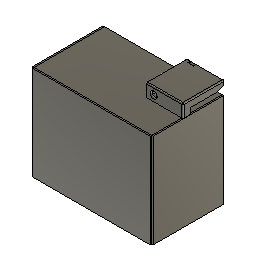
Pantry Working_ (Autodesk Fusion 360 design; units mm, degrees)
Autodesk Fusion 360 part; units mm, degrees
sketch "Sketch1" plane through (0, 0, 0) normal (0, 0, 1) x (1, 0, 0)
  line L0 (0, 0) -> (6.35, 0)
  line L1 (6.35, 0) -> (6.35, 300)
  line L2 (6.35, 300) -> (0, 300)
  line L3 (0, 300) -> (0, 0)
  line L4 (6.35, 0) -> (506.35, 0)
  line L5 (506.35, 0) -> (506.35, -6.35)
  line L6 (506.35, -6.35) -> (6.35, -6.35)
  line L7 (6.35, -6.35) -> (6.35, 0)
  line L8 (506.35, 0) -> (512.7, 0)
  line L9 (512.7, 0) -> (512.7, 300)
  line L10 (512.7, 300) -> (506.35, 300)
  line L11 (506.35, 300) -> (506.35, 0)
  line L12 (6.35, 300) -> (506.35, 300)
  dimension "d1" = 6.35
  dimension "d2" = 300
  dimension "d3" = 500
  dimension "d4" = 6.35
  dimension "d5" = 6.35
  dimension "d6" = 300
  constraint horizontal L0
  constraint vertical L1
  constraint horizontal L2
  constraint vertical L3
  constraint coincident L0.start L3.end
  constraint horizontal L4
  constraint vertical L5
  constraint horizontal L6
  constraint vertical L7
  constraint horizontal L8
  constraint vertical L9
  constraint horizontal L10
  constraint vertical L11
  measures "d1" distance of L0.start L0.end
  measures "d2" distance of L0.start L2.end
  measures "d3" distance of L0.end L4.end
  measures "d4" distance of L0.end L6.end
  measures "d5" distance of L4.end L8.end
  measures "d6" distance of L4.end L10.end
extrude "Extrude1" add sketch "Sketch1" along normal blind 400 contours L0 L1 L2 L3 | L4 L5 L6 L7 | L8 L9 L10 L11 makes body 1 at (0, 200, 133.3333)
extrude "Extrude2" add sketch "Sketch1" along normal blind 12.7 separate body contours L1 L4 L11 L12 makes body 2
ref_plane "WorkPlane1" through (0, 0, 220) normal (0, 0, 1) x (1, 0, 0)
sketch "Sketch2" plane through (0, 0, 220) normal (0, 0, 1) x (1, 0, 0)
  line L0 (6.35, 0) -> (506.35, 0)
  line L1 (506.35, 0) -> (506.35, 300)
  line L2 (506.35, 300) -> (6.35, 300)
  line L3 (6.35, 300) -> (6.35, 0)
  line L4 (6.35, 0) -> (506.35, 0)
  line L5 (506.35, 0) -> (506.35, 150)
  line L6 (506.35, 150) -> (6.35, 150)
  line L7 (6.35, 150) -> (6.35, 0)
  line L8 (506.35, 150) -> (406.35, 150)
  line L9 (406.35, 150) -> (406.35, 300)
  line L10 (406.35, 300) -> (506.35, 300)
  line L11 (506.35, 300) -> (506.35, 150)
  line L12 (6.35, 150) -> (106.35, 150)
  line L13 (106.35, 150) -> (106.35, 300)
  line L14 (106.35, 300) -> (6.35, 300)
  line L15 (6.35, 300) -> (6.35, 150)
  dimension "d12" = 500
  dimension "d13" = 150
  dimension "d14" = 100
  dimension "d15" = 150
  dimension "d16" = 100
  dimension "d17" = 150
  constraint horizontal L4
  constraint vertical L5
  constraint horizontal L6
  constraint vertical L7
  constraint coincident L0.start L3.end
  constraint horizontal L8
  constraint vertical L9
  constraint horizontal L10
  constraint vertical L11
  constraint horizontal L12
  constraint vertical L13
  constraint horizontal L14
  constraint vertical L15
  measures "d12" distance of L0.start L0.end
  measures "d13" distance of L0.start L6.end
  measures "d14" distance of L5.end L8.end
  measures "d15" distance of L5.end L1.end
  measures "d16" distance of L6.end L12.end
  measures "d17" distance of L6.end L2.end
extrude "Extrude3" add sketch "Sketch2" along normal blind 12.7 separate body contours L0 L1 L3 L4 L5 L6 L7 L8 L12 | L2 L3 L6 L12 L13 L14 L15 | L1 L2 L6 L8 L9 L10 L11 makes body 3
ref_plane "WorkPlane2" through (0, 0, 400) normal (0, 0, 1) x (1, 0, 0)
sketch "Sketch3" plane through (0, 0, 400) normal (0, 0, 1) x (1, 0, 0)
  line L0 (6.35, 0) -> (506.35, 0)
  line L1 (506.35, 0) -> (506.35, 300)
  line L2 (506.35, 300) -> (6.35, 300)
  line L3 (6.35, 300) -> (6.35, 0)
extrude "Extrude4" add sketch "Sketch3" against normal blind 12.7 separate body makes body 4
sketch "Sketch4" plane through (0, 0, 232.7) normal (0, 0, 1) x (-1, 0, 0)
  line L0 (-406.35, -150) -> (-106.35, -150)
  line L1 (-106.35, -150) -> (-106.35, -300)
  line L2 (-106.35, -300) -> (-6.35, -300)
  line L3 (-6.35, -300) -> (-6.35, 0)
  line L4 (-6.35, 0) -> (-506.35, 0)
  line L5 (-506.35, 0) -> (-506.35, -300)
  line L6 (-506.35, -300) -> (-406.35, -300)
  line L7 (-406.35, -300) -> (-406.35, -150)
  line L8 (-406.35, -150) -> (-421.35, -150)
  line L9 (-421.35, -150) -> (-421.35, -175)
  line L10 (-421.35, -175) -> (-406.35, -175)
  line L11 (-406.35, -175) -> (-406.35, -150)
  line L12 (-406.35, -150) -> (-381.35, -150)
  line L13 (-381.35, -150) -> (-381.35, -135)
  line L14 (-381.35, -135) -> (-406.35, -135)
  line L15 (-406.35, -135) -> (-406.35, -150)
  line L16 (-381.35, -150) -> (-406.35, -175)
  line L17 (-406.35, -135) -> (-421.35, -135)
  line L18 (-421.35, -135) -> (-421.35, -150)
  line L19 (-421.35, -150) -> (-406.35, -150)
  line L20 (-406.35, -150) -> (-406.35, -135)
  dimension "d23" = 15
  dimension "d24" = 25
  dimension "d25" = 25
  dimension "d26" = 15
  constraint horizontal L8
  constraint vertical L9
  constraint horizontal L10
  constraint vertical L11
  constraint coincident L0.start L7.end
  constraint horizontal L12
  constraint vertical L13
  constraint horizontal L14
  constraint vertical L15
  constraint horizontal L17
  constraint vertical L18
  constraint horizontal L19
  constraint vertical L20
  measures "d23" distance of L0.start L8.end
  measures "d24" distance of L0.start L10.end
  measures "d25" distance of L0.start L12.end
  measures "d26" distance of L0.start L14.end
extrude "Extrude5" add sketch "Sketch4" along normal blind 5 separate body contours L0 L12 L13 L14 L15 L20 | L0 L7 L11 L12 L16 | L7 L8 L9 L10 L11 L19 | L8 L15 L17 L18 L19 L20 makes body 5
extrude "Extrude7" add 1 faces at (403.0167, 158.3333, 232.7) along direction (0, 0, -1) blind 17.7 on bodies 5 bodies 5
extrude "Extrude8" cut sketch "Sketch4" against normal blind 12.7 contours L0 L12 L13 L14 L15 L20 | L7 L8 L9 L10 L11 L19 | L8 L15 L17 L18 L19 L20 bodies 5
fillet "Fillet1" radius 10 6 edges at (421.35, 175, 235.2) (421.35, 135, 235.2) (421.35, 175, 217.5) (421.35, 135, 217.5) (381.35, 135, 217.5) (381.35, 135, 235.2) on bodies 5
copy_body "Body->Comp1" bodies 1 removing the originals makes body 6 in component "walls"
copy_body "Body->Comp2" bodies 2 removing the originals makes body 7 in component "bottom"
copy_body "Body->Comp3" bodies 4 removing the originals makes body 8 in component "top"
copy_body "Body->Comp4" bodies 3 removing the originals makes body 9 in component "inner shelf"
copy_body "Body->Comp5" bodies 5 removing the originals makes body 10 in component "corner support"
sketch "Sketch5" plane through (0, 0, 400) normal (0, 0, 1) x (-1, 0, 0)
  line L0 (-6.35, -300) -> (-6.35, 0)
  line L1 (-6.35, 0) -> (-506.35, 0)
  line L2 (-506.35, 0) -> (-506.35, -300)
  line L3 (-506.35, -300) -> (-6.35, -300)
  line L4 (-506.35, -300) -> (-306.35, -300)
  line L5 (-306.35, -300) -> (-306.35, -100)
  line L6 (-306.35, -100) -> (-506.35, -100)
  line L7 (-506.35, -100) -> (-506.35, -300)
  line L8 (-506.35, -300) -> (-426.35, -300)
  line L9 (-426.35, -300) -> (-426.35, -195)
  line L10 (-426.35, -195) -> (-506.35, -195)
  line L11 (-506.35, -195) -> (-506.35, -300)
  line L12 (-426.35, -300) -> (-416.35, -300)
  line L13 (-416.35, -300) -> (-416.35, -195)
  line L14 (-416.35, -195) -> (-426.35, -195)
  line L15 (-426.35, -195) -> (-426.35, -300)
  line L16 (-416.35, -300) -> (-356.35, -300)
  line L17 (-356.35, -300) -> (-356.35, -133)
  line L18 (-356.35, -133) -> (-416.35, -133)
  line L19 (-416.35, -133) -> (-416.35, -300)
  line L20 (-356.35, -133) -> (-351.35, -133)
  line L21 (-351.35, -133) -> (-351.35, -300)
  line L22 (-351.35, -300) -> (-356.35, -300)
  line L23 (-356.35, -300) -> (-356.35, -133)
  line L24 (-351.35, -300) -> (-511.35, -300)
  line L25 (-511.35, -300) -> (-511.35, -305)
  line L26 (-511.35, -305) -> (-351.35, -305)
  line L27 (-351.35, -305) -> (-351.35, -300)
  line L28 (-511.35, -300) -> (-506.35, -300)
  line L29 (-506.35, -300) -> (-506.35, -133)
  line L30 (-506.35, -133) -> (-511.35, -133)
  line L31 (-511.35, -133) -> (-511.35, -300)
  line L32 (-351.35, -133) -> (-511.35, -133)
  line L33 (-511.35, -133) -> (-511.35, -128)
  line L34 (-511.35, -128) -> (-351.35, -128)
  line L35 (-351.35, -128) -> (-351.35, -133)
  dimension "d41" = 200
  dimension "d42" = 200
  dimension "d43" = 80
  dimension "d44" = 105
  dimension "d45" = 10
  dimension "d46" = 105
  dimension "d47" = 60
  dimension "d48" = 167
  dimension "d49" = 5
  dimension "d50" = 167
  dimension "d51" = 160
  dimension "d52" = 5
  dimension "d53" = 5
  dimension "d54" = 167
  dimension "d55" = 160
  dimension "d56" = 5
  constraint horizontal L4
  constraint vertical L5
  constraint horizontal L6
  constraint vertical L7
  constraint coincident L2.end L3.start
  constraint horizontal L8
  constraint vertical L9
  constraint horizontal L10
  constraint vertical L11
  constraint horizontal L12
  constraint vertical L13
  constraint horizontal L14
  constraint vertical L15
  constraint horizontal L16
  constraint vertical L17
  constraint horizontal L18
  constraint vertical L19
  constraint horizontal L20
  constraint vertical L21
  constraint horizontal L22
  constraint vertical L23
  constraint horizontal L24
  constraint vertical L25
  constraint horizontal L26
  constraint vertical L27
  constraint horizontal L28
  constraint vertical L29
  constraint horizontal L30
  constraint vertical L31
  constraint horizontal L32
  constraint vertical L33
  constraint horizontal L34
  constraint vertical L35
  measures "d41" distance of L2.end L4.end
  measures "d42" distance of L2.end L6.end
  measures "d43" distance of L2.end L8.end
  measures "d44" distance of L2.end L10.end
  measures "d45" distance of L8.end L12.end
  measures "d46" distance of L8.end L9.end
  measures "d47" distance of L12.end L16.end
  measures "d48" distance of L12.end L18.end
  measures "d49" distance of L17.end L20.end
  measures "d50" distance of L17.end L16.end
  measures "d51" distance of L21.end L24.end
  measures "d52" distance of L21.end L26.end
  measures "d53" distance of L24.end L2.end
  measures "d54" distance of L24.end L30.end
  measures "d55" distance of L20.end L30.end
  measures "d56" distance of L20.end L34.end
extrude "Extrude9" add sketch "Sketch5" along normal blind 55 separate body contours L3 L4 L8 L12 L16 L22 L24 L25 L26 L27 L28 | L3 L4 L17 L20 L21 L22 L23 L24 L32 | L2 L7 L18 L20 L32 L34 L35 | L2 L7 L30 L32 L33 L34 | L2 L7 L11 L24 L28 L29 L30 L31 L32 makes body 11
sketch "Sketch6" plane through (511.35, 0, 0) normal (1, 0, 0) x (0, 1, 0)
  line L0 (128, 400) -> (305, 400)
  line L1 (305, 400) -> (305, 455)
  line L2 (305, 455) -> (128, 455)
  line L3 (128, 455) -> (128, 400)
  line L4 (305, 400) -> (160, 400)
  line L5 (160, 400) -> (160, 425)
  line L6 (160, 425) -> (305, 425)
  line L7 (305, 425) -> (305, 400)
  dimension "d59" = 145
  dimension "d60" = 25
  constraint horizontal L4
  constraint vertical L5
  constraint horizontal L6
  constraint vertical L7
  constraint coincident L0.end L1.start
  measures "d59" distance of L0.end L4.end
  measures "d60" distance of L0.end L6.end
sketch "Sketch7" plane through (0, 305, 0) normal (0, 1, 0) x (-1, 0, 0)
  line L0 (-511.35, 400) -> (-351.35, 400)
  line L1 (-351.35, 400) -> (-351.35, 455)
  line L2 (-351.35, 455) -> (-511.35, 455)
  line L3 (-511.35, 455) -> (-511.35, 400)
  line L4 (-511.35, 400) -> (-461.35, 400)
  line L5 (-461.35, 400) -> (-461.35, 435)
  line L6 (-461.35, 435) -> (-511.35, 435)
  line L7 (-511.35, 435) -> (-511.35, 400)
  line L8 (-351.35, 400) -> (-376.35, 400) construction
  line L9 (-376.35, 400) -> (-389.35, 400)
  line L10 (-389.35, 400) -> (-389.35, 422)
  line L11 (-389.35, 422) -> (-376.35, 422)
  line L12 (-376.35, 422) -> (-376.35, 400)
  line L13 (-445, 440) -> (-420, 440)
  line L14 (-420, 440) -> (-420, 425)
  line L15 (-420, 425) -> (-445, 425)
  line L16 (-445, 425) -> (-445, 440)
  dimension "d61" = 50
  dimension "d62" = 35
  dimension "d63" = 25
  dimension "d64" = 13
  dimension "d65" = 22
  dimension "d66" = 25
  dimension "d67" = 15
  constraint horizontal L4
  constraint vertical L5
  constraint horizontal L6
  constraint vertical L7
  constraint coincident L0.start L3.end
  constraint coincident L0.end L1.start
  constraint perpendicular L1 L8
  constraint horizontal L9
  constraint vertical L10
  constraint horizontal L11
  constraint vertical L12
  constraint horizontal L13
  constraint vertical L14
  constraint horizontal L15
  constraint vertical L16
  measures "d61" distance of L0.start L4.end
  measures "d62" distance of L0.start L6.end
  measures "d63" distance of L0.end L8.end
  measures "d64" distance of L8.end L9.end
  measures "d65" distance of L8.end L11.end
  measures "d66" distance of L13.start L13.end
  measures "d67" distance of L13.start L15.end
sketch "Sketch8" plane through (0, 128, 0) normal (0, -1, 0) x (1, 0, 0)
  line L0 (351.35, 400) -> (511.35, 400)
  line L1 (511.35, 400) -> (511.35, 455)
  line L2 (511.35, 455) -> (351.35, 455)
  line L3 (351.35, 455) -> (351.35, 400)
  line L4 (351.35, 400) -> (386.35, 400) construction
  line L5 (386.35, 400) -> (386.35, 425) construction
  line L6 (386.35, 425) -> (351.35, 425) construction
  line L7 (351.35, 425) -> (351.35, 400) construction
  circle A0 centre (386.35, 425) radius 10
  dimension "d68" = 35
  dimension "d69" = 25
  dimension "d70" = 20
  constraint horizontal L4
  constraint vertical L5
  constraint horizontal L6
  constraint vertical L7
  constraint coincident L0.start L3.end
  constraint coincident L5.end L6.start
  measures "d68" distance of L0.start L4.end
  measures "d69" distance of L0.start L6.end
  measures "d70" diameter of A0
extrude "Extrude10" cut sketch "Sketch8" against normal blind 5 contours A0 bodies 11
extrude "Extrude11" cut sketch "Sketch7" against normal blind 5 contours L0 L3 L4 L5 L6 L7 | L0 L9 L10 L11 L12 | L13 L14 L15 L16 bodies 11
chamfer "Chamfer1" distance 7 distance2 4 4 edges at (445, 305, 432.5) (432.5, 305, 440) (420, 305, 432.5) (432.5, 305, 425) measured on face at (423.5667, 305, 408.3333) measured on face at (423.5667, 305, 408.3333) measured on face at (423.5667, 305, 408.3333) measured on face at (423.5667, 305, 408.3333) on bodies 11
extrude "Extrude12" cut sketch "Sketch6" against normal blind 5 contours L0 L1 L4 L5 L6 L7 bodies 11
chamfer "Chamfer2" distance 10 distance2 30 1 edges at (508.85, 300, 425) measured on face at (509.6833, 300, 431.6667) on bodies 11
sketch "Sketch9" plane through (0, 0, 455) normal (0, 0, 1) x (-1, 0, 0)
  line L0 (-356.35, -300) -> (-506.35, -300)
  line L1 (-506.35, -300) -> (-506.35, -133)
  line L2 (-506.35, -133) -> (-356.35, -133)
  line L3 (-356.35, -133) -> (-356.35, -300)
  line L4 (-511.35, -128) -> (-511.35, -305)
  line L5 (-511.35, -305) -> (-351.35, -305)
  line L6 (-351.35, -305) -> (-351.35, -128)
  line L7 (-351.35, -128) -> (-511.35, -128)
  line L8 (-370, -300) -> (-395, -300)
  line L9 (-395, -300) -> (-395, -290)
  line L10 (-395, -290) -> (-370, -290)
  line L11 (-370, -290) -> (-370, -300)
  dimension "d83" = 25
  dimension "d84" = 10
  constraint horizontal L8
  constraint vertical L9
  constraint horizontal L10
  constraint vertical L11
  constraint coincident L0 L8.start
  measures "d83" distance of L8.start L8.end
  measures "d84" distance of L8.start L10.end
extrude "Extrude13" add sketch "Sketch9" against normal blind 5 contours L0 L1 L2 L3 L9 L10 L11 bodies 11
fillet "Fillet2" radius 5 8 edges at (511.35, 216.5, 455) (511.35, 128, 427.5) (431.35, 128, 455) (351.35, 216.5, 455) (431.35, 305, 455) (351.35, 305, 427.5) (511.35, 305, 445) (351.35, 128, 427.5) on bodies 11
fillet "Fillet3" radius 5 4 edges at (452, 305, 432.5) (432.5, 305, 418) (432.5, 305, 447) (413, 305, 432.5) on bodies 11
fillet "Fillet4" radius 14 8 edges at (452.0445, 304.8325, 417.9555) (447.9236, 302.6706, 422.0764) (452.0445, 304.8325, 447.0445) (447.9236, 302.6706, 442.9236) (412.9555, 304.8325, 447.0445) (417.0764, 302.6706, 442.9236) (417.0764, 302.6706, 422.0764) (412.9555, 304.8325, 417.9555) on bodies 11
fillet "Fillet5" radius 5 1 edges at (377.0267, 128, 428.6162) on bodies 11
copy_body "Body->Comp6" bodies 11 removing the originals makes body 12 in component "Component"
component "walls" placed x (1, 0, 0) y (0, 1, 0) z (0, 0, 1) at (0, 0, 0)
component "bottom" placed x (1, 0, 0) y (0, 1, 0) z (0, 0, 1) at (0, 0, 0)
component "top" placed x (1, 0, 0) y (0, 1, 0) z (0, 0, 1) at (0, 0, 0)
component "inner shelf" placed x (1, 0, 0) y (0, 1, 0) z (0, 0, 1) at (0, 0, 0)
component "corner support" placed x (1, 0, 0) y (0, 1, 0) z (0, 0, 1) at (0, 0, 0)
component "corner support" placed x (0, -1, 0) y (1, 0, 0) z (0, 0, 1) at (-43.65, 556.35, 0)
component "Component" placed x (1, 0, 0) y (0, 1, 0) z (0, 0, 1) at (0, 0, 0)
equation "d1 = ( 1 / 4 ) * 1 in"
equation "d4 = 1 / 4 * 1 in"
equation "d5 = 1 / 4 * 1 in"
equation "d9 = 1 / 2 * 1 in"
equation "d18 = 1 / 2 * 1 in"
equation "d21 = -1 / 2 * 1 in"
equation "d31 = 1.27 cm + 0.5 cm"
named bodies: "walls", "bottom", "inner shelf", "top", "corner support"
